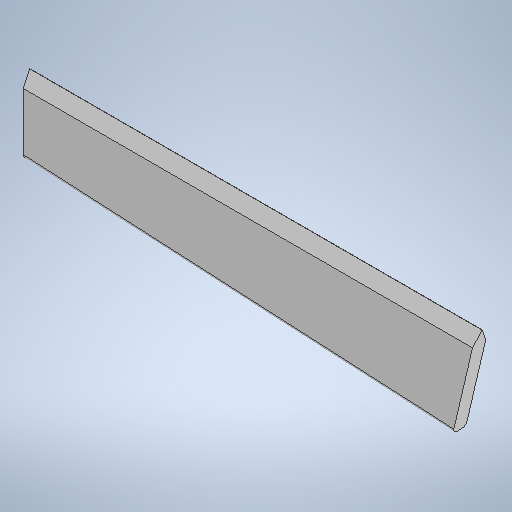
# Autodesk Inventor part: Part11
Saved by Autodesk Inventor 2025.3 (Build 293356000, 356)
## iProperties
Created: 2025-07-09
Part Number: Part11
Material: Generic
Document SubType Name: Modeling
Designer: steve
Density: 1 g/cm^3
Appearance: Default
Author: steve
Autodesk Inventor part; units mm, degrees
ref_plane "YZ Plane" through (0, 0, 0) normal (1, 0, 0) x (0, 1, 0)
ref_plane "XZ Plane" through (0, 0, 0) normal (0, 1, 0) x (-1, 0, 0)
ref_plane "XY Plane" through (0, 0, 0) normal (0, 0, 1) x (1, 0, 0)
sketch "Sketch1" plane through (0, 0, 0) normal (0, 0, 1) x (1, 0, 0)
  line L0 (-23.2595, -28.4822) -> (192.7405, -28.4822)
  line L1 (-23.2595, -28.4822) -> (-13.2595, -28.4822)
  line L2 (-13.2595, -28.4822) -> (-3.2595, -28.4822)
  line L3 (-3.2595, -28.4822) -> (-3.2595, -71.1622)
  line L4 (-23.2595, -28.4822) -> (183.7405, -28.4822)
  line L5 (183.7405, -28.4822) -> (183.7405, -61.4022)
  line L6 (183.7405, -61.4022) -> (-3.2595, -71.1622)
  line L7 (-13.2595, -28.4822) -> (-3.2595, -71.1622)
  line L8 (183.7405, -28.4822) -> (183.7405, 26.1278)
  line L9 (-23.2595, -28.4822) -> (-23.2595, 82.8078)
  line L10 (-23.2595, 82.8078) -> (183.7405, 26.1278)
  line L11 (183.7405, 26.1278) -> (183.7405, 27.1278)
  line L12 (183.7405, 27.1278) -> (192.7405, 24.6634)
  line L13 (192.7405, -28.4822) -> (192.7405, 24.6634)
  line L14 (183.7405, -61.4022) -> (192.7405, -60.9325)
  line L15 (192.7405, -28.4822) -> (192.7405, -60.9325)
  line L16 (-23.2595, -28.4822) -> (-33.2595, -28.4822)
  line L17 (-33.2595, -28.4822) -> (-43.2595, -28.4822)
  line L18 (-23.2595, -28.4822) -> (-230.2595, -28.4822)
  line L19 (-230.2595, -28.4822) -> (-230.2595, -61.4022)
  line L20 (-43.2595, -28.4822) -> (-43.2595, -71.1622)
  line L21 (-230.2595, -61.4022) -> (-43.2595, -71.1622)
  line L22 (-33.2595, -28.4822) -> (-43.2595, -71.1622)
  line L23 (-239.2595, -28.4822) -> (-239.2595, -60.9325)
  line L24 (-230.2595, -61.4022) -> (-239.2595, -60.9325)
  line L25 (-23.2595, -28.4822) -> (-239.2595, -28.4822)
  line L26 (-239.2595, -28.4822) -> (-239.2595, 24.6634)
  line L27 (-230.2595, 27.1278) -> (-239.2595, 24.6634)
  line L28 (-230.2595, -28.4822) -> (-230.2595, 26.1278)
  line L29 (-230.2595, 26.1278) -> (-230.2595, 27.1278)
  line L30 (-23.2595, 82.8078) -> (-230.2595, 26.1278)
  point P0 (0, 0)
  dimension "d0" = 216
  dimension "d1" = 10
  dimension "d2" = 10
  dimension "d3" = 42.68
  dimension "d4" = 207
  dimension "d5" = 32.92
  dimension "d6" = 54.61
  dimension "d7" = 111.29
  dimension "d8" = 1
  constraints: 62 end point, 10 symmetric about line, 7 vertical, 6 point on line, 1 collinear, 1 horizontal, 1 parallel
  measures "d0" distance of L9.start L15.start
  measures "d1" distance of L9.start L7.start
  measures "d2" distance of L7.start L3.start
  measures "d3" distance of L3.start L6.end
  measures "d4" distance of L9.start L5.start
  measures "d5" distance of L5.start L14.start
  measures "d6" distance of L5.start L8.end
  measures "d7" distance of L9.start L9.end
  measures "d8" distance of L8.end L11.end
extrude "Extrusion1" add sketch "Sketch1" along normal mid plane 5.7 contours L22 L20 L17 | L20 L21 L19 L18
chamfer "Chamfer1" distance 6 angle 25 1 edges at (-131.7595, -28.4822, -2.85) measured on face at (-102.2595, -42.7089, -2.85)
fillet "Fillet1" radius 2 2 edges at (-136.7595, -66.2822, -2.85) (-136.7595, -66.2822, 2.85)
chamfer "Chamfer2" distance 6 angle 25 1 edges at (-131.7595, -28.4822, 2.85) measured on face at (-102.105, -42.0494, 2.85)
body "Solid1"
